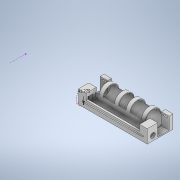
# Autodesk Inventor part: front_2-6
Saved by Autodesk Inventor 2020 (Build 240168000, 168)
## iProperties
Created: 2020-02-06
Part Number: front_2-6
Material: Generic
Document SubType Name: Modeling
Designer: akend
Density: 1 g/cm^3
Appearance: Default
Author: akend
## iProperties of the stored document _3DPrint.ipt
Created: 2020-02-07
Part Number: _3DPrint
Material: Generic
Document SubType Name: Modeling
Designer: akend
Density: 1 g/cm^3
Appearance: Default
Author: akend
Autodesk Inventor part; units mm, degrees
ref_plane "YZ Plane" through (0, 0, 0) normal (1, 0, 0) x (0, 1, 0)
ref_plane "XZ Plane" through (0, 0, 0) normal (0, 1, 0) x (-1, 0, 0)
sketch "Sketch1" plane through (0, 0, 0) normal (1, 0, 0) x (0, 1, 0)
  line L0 (0, 0) -> (35, 0)
  line L1 (35, 0) -> (35, 27)
  line L2 (35, 27) -> (0, 27)
  line L3 (0, 27) -> (0, 0)
  line L4 (0, 27) -> (25, 27) construction
  line L5 (25, 27) -> (25, 0) construction
  line L6 (25, 0) -> (0, 0) construction
  line L7 (0, 0) -> (0, 27) construction
  circle A0 centre (12.5, 12.5) radius 6.35
  dimension "d0" = 35
  dimension "d1" = 27
  dimension "d2" = 25
  dimension "d3" = 12.7
  constraints: 16 end point, 4 parallel, 2 horizontal, 2 perpendicular, 1 centre point, 1 coincident, 1 point on line
  measures "d0" distance of L2.end L1.end
  measures "d1" distance of L1.end L0.end
  measures "d2" distance of L5.end L6.end
  measures "d3" diameter of A0
extrude "Extrusion1" add sketch "Sketch1" along normal blind 10
sketch "Sketch2" plane through (10, 0, 0) normal (1, 0, 0) x (0, 0, -1)
  line L0 (0, 35) -> (-27, 35) projected
  line L1 (0, 0) -> (0, 35) projected
  line L2 (-27, 35) -> (0, 35)
  line L3 (0, 35) -> (0, 25)
  line L4 (0, 25) -> (-27, 25)
  line L5 (-27, 25) -> (-27, 35)
  dimension "d6" = 10
  constraints: 8 end point, 2 parallel, 1 horizontal, 1 perpendicular, 1 point on line
  measures "d6" distance of L2.end L3.end
extrude "Extrusion2" add sketch "Sketch2" along normal blind 10
sketch "Sketch3" plane through (10, 0, 0) normal (1, 0, 0) x (0, 0, -1)
  point P0 (0, 0)
sketch "Sketch4" plane through (0, 0, 0) normal (0, 0, -1) x (-1, 0, 0)
  point P0 (0, 0)
sketch "Sketch5" plane through (10, 0, 0) normal (1, 0, 0) x (0, 0, -1)
  point P0 (0, 0)
sketch "Sketch6" plane through (10, 0, 0) normal (1, 0, 0) x (0, 0, -1)
  line L0 (-27, 25) -> (-27, 0) projected
  line L1 (-27, 0) -> (-22, 0)
  line L2 (-22, 0) -> (-22, 11)
  line L3 (-22, 11) -> (-27, 11)
  line L4 (-27, 11) -> (-27, 0)
  line L5 (-22, 14) -> (-27, 14)
  line L6 (-27, 14) -> (-27, 19)
  line L7 (-27, 19) -> (-22, 19)
  line L8 (-22, 19) -> (-22, 14)
  point P0 (0, 0)
  dimension "d9" = 5
  dimension "d10" = 11
  dimension "d11" = 5
  constraints: 16 end point, 4 parallel, 2 horizontal, 2 perpendicular, 2 point on line
  measures "d9" distance of L3.end L2.end
  measures "d10" distance of L2.end L1.end
  measures "d11" distance of L5.end L6.end
extrude "Extrusion3" add sketch "Sketch6" along normal blind 150
sketch "Sketch7" plane through (10, 19, 27) normal (0, 1, 0) x (1, 0, 0)
  line L0 (-10, 0) -> (10, 0) projected
  line L1 (0, 5) -> (150, 5) projected
  line L2 (0, 0) -> (10, 0)
  line L3 (10, 0) -> (10, 5)
  line L4 (10, 5) -> (0, 5)
  line L5 (0, 5) -> (0, 0)
  point P0 (-10, 27)
  dimension "d14" = 10
  constraints: 8 end point, 2 parallel, 1 horizontal, 1 midpoint, 1 perpendicular, 1 point on line
  measures "d14" distance of L4.end L3.end
extrude "Extrusion4" add sketch "Sketch7" along normal blind 7.5
sketch "Sketch8" plane through (160, 0, 0) normal (1, 0, 0) x (0, 0, -1)
  line L0 (-27, 14) -> (-22, 14) projected
  line L1 (-27, 14) -> (-22, 14)
  line L2 (-22, 25) -> (-22, 14) projected
  line L3 (-22, 14) -> (-22, 25)
  line L4 (-22, 25) -> (0, 25) projected
  line L5 (-22, 25) -> (0, 25)
  line L6 (0, 25) -> (0, 35) projected
  line L7 (0, 25) -> (0, 35)
  line L8 (0, 35) -> (-27, 35)
  line L9 (-27, 35) -> (-27, 14)
  line L10 (-22, 11) -> (-22, 0) projected
  line L11 (-27, 0) -> (-22, 0)
  line L12 (-22, 0) -> (-22, 11)
  line L13 (-22, 11) -> (-27, 11)
  line L14 (-27, 11) -> (-27, 0)
  point P0 (0, 0)
  constraints: 20 end point, 5 perpendicular, 4 equal length, 1 horizontal
extrude "Extrusion5" add sketch "Sketch8" along normal blind 10
sketch "Sketch9" plane through (170, 0, 0) normal (1, 0, 0) x (0, 0, -1)
  line L0 (0, 35) -> (-27, 35) projected
  line L1 (-27, 35) -> (0, 35)
  line L2 (0, 35) -> (0, 0)
  line L3 (0, 0) -> (-27, 0)
  line L4 (-27, 0) -> (-27, 35)
  circle A0 centre (-12.5, 12.5) radius 6.35 projected
  circle A1 centre (-12.5, 12.5) radius 6.35
  constraints: 8 end point, 2 parallel, 1 centre point, 1 coincident, 1 horizontal, 1 perpendicular
extrude "Extrusion6" add sketch "Sketch9" along normal blind 10
fillet "Fillet1" radius 2 2 edges at (90, 11, 22) (90, 14, 22)
sketch "Sketch10" plane through (20, 0, 0) normal (1, 0, 0) x (0, 0, -1)
  line L0 (0, 35) -> (-27, 35) projected
  line L1 (-13.5, 35) -> (-20.5, 35)
  line L2 (-20.5, 35) -> (-6.5, 35)
  line L3 (-20.5, 35) -> (-6.5, 35)
  line L4 (-6.5, 35) -> (-6.5, 32)
  line L5 (-6.5, 32) -> (-20.5, 32)
  line L6 (-20.5, 32) -> (-20.5, 35)
  point P0 (0, 0)
  dimension "d22" = 7
  dimension "d23" = 14
  dimension "d24" = 3
  constraints: 12 end point, 2 parallel, 2 point on line, 1 horizontal, 1 midpoint, 1 perpendicular
  measures "d22" distance of L1.start L1.end
  measures "d23" distance of L1.end L2.end
  measures "d24" distance of L3.end L4.end
extrude "Extrusion7" add sketch "Sketch10" along normal blind 140
sketch "Sketch11" plane through (0, 35, 27) normal (0, 1, 0) x (1, 0, 0)
  point P0 (0, 27)
sketch "Sketch12" plane through (160, 25, 0) normal (0, 0, -1) x (-1, 0, 0)
  line L0 (-4, 3.5) -> (-16, 3.5)
  line L1 (-16, 3.5) -> (-16, 6.5)
  line L2 (-16, 6.5) -> (-4, 6.5)
  line L3 (-4, 6.5) -> (-4, 3.5)
  line L4 (-4, 3.5) -> (-16, 6.5) construction
  line L5 (-16, 3.5) -> (-4, 6.5) construction
  line L6 (156, 6.5) -> (144, 6.5)
  line L7 (144, 6.5) -> (144, 3.5)
  line L8 (144, 3.5) -> (156, 3.5)
  line L9 (156, 3.5) -> (156, 6.5)
  line L10 (156, 6.5) -> (144, 3.5) construction
  line L11 (144, 6.5) -> (156, 3.5) construction
  point P0 (160, -25)
  point P1 (-10, 5)
  point P2 (150, 5)
  dimension "d27" = 12
  dimension "d28" = 3
  dimension "d29" = 12
  dimension "d30" = 3
  constraints: 24 end point, 4 midpoint, 4 parallel, 2 horizontal, 2 perpendicular
  measures "d27" distance of L0.start L0.end
  measures "d28" distance of L0.end L1.end
  measures "d29" distance of L6.start L6.end
  measures "d30" distance of L7.end L6.end
extrude "Extrusion8" cut sketch "Sketch12" against normal blind 23.5
sketch "Sketch13" plane through (0, 0, 0) normal (-1, 0, 0) x (0, 0, 1)
  circle A0 centre (12.5, 12.5) radius 6.35 construction
  circle A1 centre (12.5, 12.5) radius 20.6375 construction
  point P0 (0, 0)
  dimension "d33" = 41.275
  constraints: 1 centre point, 1 coincident
  measures "d33" diameter of A1
sketch "Sketch14" plane through (170, 0, 0) normal (-1, 0, 0) x (0, 0, 1)
  circle A0 centre (12.5, 12.5) radius 6.35 projected
  circle A1 centre (12.5, 12.5) radius 6.35
  circle A2 centre (12.5, 12.5) radius 3.5
  point P0 (0, 0)
  dimension "d34" = 7
  constraints: 2 centre point, 2 coincident
  measures "d34" diameter of A2
extrude "Extrusion9" add sketch "Sketch14" against normal blind 4.5
sketch "Sketch15" plane through (10, 0, 0) normal (1, 0, 0) x (0, 0, -1)
  circle A0 centre (-12.5, 12.5) radius 3.5 projected
  circle A1 centre (-12.5, 12.5) radius 6.35
  circle A2 centre (-12.5, 12.5) radius 3.5
  point P0 (0, 0)
  dimension "d37" = 7
  constraints: 2 centre point, 2 coincident
  measures "d37" diameter of A2
extrude "Extrusion10" add sketch "Sketch15" against normal blind 4.5
sketch "Sketch16" plane through (0, 0, 27) normal (0, 0, 1) x (1, 0, 0)
  point P0 (0, 0)
sketch "Sketch17" plane through (0, 0, 27) normal (0, 0, 1) x (1, 0, 0)
  point P0 (0, 0)
sketch "Sketch18" plane through (0, 0, 27) normal (0, 0, 1) x (1, 0, 0)
  line L0 (0, 35) -> (0, 0) projected
  line L1 (180, 35) -> (180, 0) projected
  line L2 (0, 0) -> (180, 0)
  line L3 (180, 0) -> (180, 3)
  line L4 (180, 3) -> (0, 3)
  line L5 (0, 3) -> (0, 0)
  point P0 (0, 3)
  dimension "d40" = 3
  constraints: 8 end point, 2 parallel, 1 horizontal, 1 perpendicular, 1 point on line
  measures "d40" distance of L3.end L2.end
extrude "Extrusion11" add sketch "Sketch18" against normal blind 67
sketch "Sketch19" plane through (0, 3, 27) normal (0, 1, 0) x (-1, 0, 0)
  line L0 (180, 0) -> (180, -42) construction
  point P0 (0, 0)
  constraints: 2 end point
sketch "Sketch20" plane through (0, 3, -40) normal (0, 1, 0) x (1, 0, 0)
  circle A0 centre (90, -20) radius 19
  circle A1 centre (90, -20) radius 20
  circle A2 centre (50, -20) radius 20
  circle A3 centre (50, -20) radius 19
  circle A4 centre (130, -20) radius 20
  circle A5 centre (130, -20) radius 19
  point P0 (0, -40)
  point P1 (110, -20)
  point P2 (70, -20)
  dimension "d43" = 38
  dimension "d44" = 38
  dimension "d45" = 38
  constraints: 6 centre point, 4 coincident, 2 equal radius
  measures "d43" diameter of A0
  measures "d44" diameter of A3
  measures "d45" diameter of A5
extrude "Extrusion12" add sketch "Sketch20" along normal blind 30
sketch "Sketch21" plane through (10, 3, 22) normal (0, 1, 0) x (1, 0, 0)
  line L0 (-10, 22) -> (-10, 62) projected
  line L1 (-10, 62) -> (10, 62)
  line L2 (10, 62) -> (10, 52)
  line L3 (10, 52) -> (-10, 52)
  line L4 (-10, 52) -> (-10, 62)
  line L5 (170, 62) -> (-10, 62) projected
  line L6 (170, 62) -> (150, 62)
  line L7 (150, 62) -> (150, 52)
  line L8 (150, 52) -> (170, 52)
  line L9 (170, 52) -> (170, 62)
  dimension "d48" = 10
  dimension "d49" = 10
  constraints: 16 end point, 4 parallel, 2 horizontal, 2 perpendicular
  measures "d48" distance of L1.end L2.end
  measures "d49" distance of L7.end L6.end
extrude "Extrusion13" add sketch "Sketch21" along normal blind 32
sketch "Sketch22" plane through (4, 28.5, 0) normal (0, 1, 0) x (1, 0, 0)
  point P0 (-4, 0)
sketch "Sketch23" plane through (0, 0, -40) normal (0, 0, -1) x (-1, 0, 0)
  line L0 (-4, 28.5) -> (-16, 28.5) projected
  line L1 (-4, 31.5) -> (-4, 28.5) projected
  line L2 (-16, 28.5) -> (-4, 28.5)
  line L3 (-4, 28.5) -> (-4, 31.5)
  line L4 (-4, 31.5) -> (-16, 31.5)
  line L5 (-16, 31.5) -> (-16, 28.5)
  line L6 (-164, 28.5) -> (-176, 28.5) projected
  line L7 (-164, 31.5) -> (-164, 28.5) projected
  line L8 (-176, 28.5) -> (-164, 28.5)
  line L9 (-164, 28.5) -> (-164, 31.5)
  line L10 (-164, 31.5) -> (-176, 31.5)
  line L11 (-176, 31.5) -> (-176, 28.5)
  point P0 (0, 0)
  constraints: 16 end point, 4 parallel, 2 horizontal, 2 perpendicular
extrude "Extrusion14" cut sketch "Sketch23" against normal blind 10
sketch "Sketch24" plane through (130, 33, -20) normal (0, 1, 0) x (1, 0, 0)
  line L0 (27.2959, -23.1323) -> (-103.8128, -23.1323)
  line L1 (-103.8128, -23.1323) -> (-103.8128, 25.7271)
  line L2 (-103.8128, 25.7271) -> (27.2959, 25.7271)
  line L3 (27.2959, 25.7271) -> (27.2959, -23.1323)
  point P0 (-130, -20)
  constraints: 8 end point, 2 parallel, 1 horizontal, 1 perpendicular
extrude "Extrusion15" cut sketch "Sketch24" against normal blind 30
sketch "Sketch25" plane through (10, 3, 22) normal (0, 1, 0) x (1, 0, 0)
  circle A0 centre (80, 38.75) radius 19
  circle A1 centre (80, 38.75) radius 20.75
  circle A2 centre (121.5, 38.75) radius 20.75
  circle A3 centre (121.5, 38.75) radius 19
  circle A4 centre (38.5, 38.75) radius 20.75
  circle A5 centre (38.5, 38.75) radius 19
  point P0 (-10, 22)
  point P1 (59.25, 38.75)
  point P2 (100.75, 38.75)
  dimension "d56" = 38
  dimension "d57" = 41.5
  dimension "d58" = 38
  dimension "d59" = 38
  constraints: 6 centre point, 3 coincident, 2 equal radius
  measures "d56" diameter of A0
  measures "d57" diameter of A1
  measures "d58" diameter of A3
  measures "d59" diameter of A5
extrude "Extrusion16" add sketch "Sketch25" along normal blind 45
sketch "Sketch26" plane through (0, 35, 27) normal (0, 1, 0) x (1, 0, 0)
  line L0 (20, 6.5) -> (160, 6.5) projected
  line L1 (20, 20.5) -> (160, 20.5) projected
  line L2 (20, 6.5) -> (160, 6.5)
  line L3 (160, 6.5) -> (160, 20.5)
  line L4 (160, 20.5) -> (20, 20.5)
  line L5 (20, 20.5) -> (20, 6.5)
  point P0 (0, 27)
  constraints: 8 end point, 2 parallel, 1 horizontal, 1 perpendicular
extrude "Extrusion17" cut sketch "Sketch26" against normal blind 5
sketch "Sketch27" plane through (10, 48, 22) normal (0, 1, 0) x (1, 0, 0)
  line L0 (16.1578, 67.5748) -> (146.5005, 67.5748)
  line L1 (146.5005, 67.5748) -> (146.5005, 15.2049)
  line L2 (146.5005, 15.2049) -> (16.1578, 15.2049)
  line L3 (16.1578, 15.2049) -> (16.1578, 67.5748)
  point P0 (-10, 22)
  constraints: 8 end point, 2 parallel, 1 horizontal, 1 perpendicular
extrude "Extrusion18" cut sketch "Sketch27" against normal blind 45
sketch "Sketch28" plane through (10, 3, 22) normal (0, 1, 0) x (1, 0, 0)
  point P0 (-10, 22)
sketch "Sketch29" plane through (0, 0, 0) normal (-1, 0, 0) x (0, 0, 1)
  point P0 (0, 0)
sketch "Sketch30" plane through (20, 3, -30) normal (1, 0, 0) x (0, 0, -1)
  circle A0 centre (-12, 19) radius 19
  line L0 (-30, 0) -> (0, 0) projected
  circle A1 centre (-12, 19) radius 20.75
  point P0 (-30, -3)
  point P1 (-3.6596, 0)
  point P2 (-20.3404, 0)
  point P3 (-12, 0)
  dimension "d66" = 41.5
  constraints: 2 centre point, 1 coincident, 1 tangent
  measures "d66" diameter of A1
extrude "Extrusion19" add sketch "Sketch30" along normal blind 140 contours L0 A1 picked at (-31.4706, 19.7749)
ref_plane "Work Plane1" through (20, 42.75, -18) normal (0, 1, 0) x (-1, 0, 0)
sketch "Sketch31" plane through (20, 42.75, -18) normal (0, 1, 0) x (-1, 0, 0)
  line L0 (0, -22) -> (-140, -22) projected
  line L1 (0, 20.75) -> (-140, 20.75) projected
  line L2 (-140, -22) -> (-130, -22)
  line L3 (-130, -22) -> (-130, 20.75)
  line L4 (-130, 20.75) -> (-140, 20.75)
  line L5 (-140, 20.75) -> (-140, -22)
  line L6 (-130, 20.75) -> (-120, 20.75)
  line L7 (-120, 20.75) -> (-120, -22)
  line L8 (-120, -22) -> (-130, -22)
  line L9 (-130, -22) -> (-130, 20.75)
  line L10 (-120, 20.75) -> (-110, 20.75)
  line L11 (-110, 20.75) -> (-110, -22)
  line L12 (-110, -22) -> (-120, -22)
  line L13 (-120, -22) -> (-120, 20.75)
  line L14 (-110, 20.75) -> (-100, 20.75)
  line L15 (-100, 20.75) -> (-100, -22)
  line L16 (-100, -22) -> (-110, -22)
  line L17 (-110, -22) -> (-110, 20.75)
  line L18 (-100, 20.75) -> (-90, 20.75)
  line L19 (-90, 20.75) -> (-90, -22)
  line L20 (-90, -22) -> (-100, -22)
  line L21 (-100, -22) -> (-100, 20.75)
  line L22 (-90, 20.75) -> (-80, 20.75)
  line L23 (-80, 20.75) -> (-80, -22)
  line L24 (-80, -22) -> (-90, -22)
  line L25 (-90, -22) -> (-90, 20.75)
  line L26 (-80, 20.75) -> (-70, 20.75)
  line L27 (-70, 20.75) -> (-70, -22)
  line L28 (-70, -22) -> (-80, -22)
  line L29 (-80, -22) -> (-80, 20.75)
  line L30 (-70, 20.75) -> (-60, 20.75)
  line L31 (-60, 20.75) -> (-60, -22)
  line L32 (-60, -22) -> (-70, -22)
  line L33 (-70, -22) -> (-70, 20.75)
  line L34 (-60, 20.75) -> (-50, 20.75)
  line L35 (-50, 20.75) -> (-50, -22.9756)
  line L36 (-50, -22.9756) -> (-60, -22.9756)
  line L37 (-60, -22.9756) -> (-60, 20.75)
  line L38 (-50, 20.75) -> (-40, 20.75)
  line L39 (-40, 20.75) -> (-40, -22)
  line L40 (-40, -22) -> (-50, -22)
  line L41 (-50, -22) -> (-50, 20.75)
  line L42 (-40, 20.75) -> (-30, 20.75)
  line L43 (-30, 20.75) -> (-30, -22)
  line L44 (-30, -22) -> (-40, -22)
  line L45 (-40, -22) -> (-40, 20.75)
  line L46 (-30, 20.75) -> (-20, 20.75)
  line L47 (-20, 20.75) -> (-20, -22)
  line L48 (-20, -22) -> (-30, -22)
  line L49 (-30, -22) -> (-30, 20.75)
  line L50 (-20, 20.75) -> (-10, 20.75)
  line L51 (-10, 20.75) -> (-10, -22)
  line L52 (-10, -22) -> (-20, -22)
  line L53 (-20, -22) -> (-20, 20.75)
  line L54 (-10, 20.75) -> (0, 20.75)
  line L55 (0, 20.75) -> (0, -22)
  line L56 (0, -22) -> (-10, -22)
  line L57 (-10, -22) -> (-10, 20.75)
  point P0 (20, 18)
  point P1 (-80, -22)
  point P2 (-60, -22)
  point P3 (-20, -22)
  point P4 (-10, -22)
  point P5 (-120, -22)
  point P6 (-90, -22)
  dimension "d69" = 10
  dimension "d70" = 10
  dimension "d71" = 10
  dimension "d72" = 10
  dimension "d73" = 10
  dimension "d74" = 10
  dimension "d75" = 10
  dimension "d76" = 10
  dimension "d77" = 10
  dimension "d78" = 10
  dimension "d79" = 10
  dimension "d80" = 10
  dimension "d81" = 10
  constraints: 112 end point, 28 parallel, 14 horizontal, 14 perpendicular, 12 point on line
  measures "d69" distance of L4.end L3.end
  measures "d70" distance of L7.end L8.end
  measures "d71" distance of L11.end L12.end
  measures "d72" distance of L15.end L16.end
  measures "d73" distance of L19.end L20.end
  measures "d74" distance of L23.end L24.end
  measures "d75" distance of L27.end L28.end
  measures "d76" distance of L31.end L32.end
  measures "d77" distance of L35.end L36.end
  measures "d78" distance of L39.end L40.end
  measures "d79" distance of L43.end L44.end
  measures "d80" distance of L47.end L48.end
  measures "d81" distance of L51.end L52.end
extrude "Extrusion20" cut sketch "Sketch31" against normal blind 19 contours L0 L51 L1 L55 | L0 L43 L1 L47 | L0 L39 L1 L43 | L0 L35 L1 L39 | L0 L27 L1 L31 | L0 L23 L1 L27 | L0 L15 L1 L19 | L0 L11 L1 L15 | L0 L7 L1 L11 | L0 L5 L1 L3
body "Solid1"
